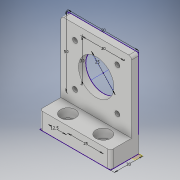
# Autodesk Inventor part: mirror-bracket
Saved by Autodesk Inventor 2017 (Build 210142000, 142)
## iProperties
Created: 2022-08-02
Part Number: mirror-bracket
Material: Generic
Document SubType Name: Modeling
Designer: Nikita
Density: 1 g/cm^3
Appearance: Default
Author: Nikita
Autodesk Inventor part; units mm, degrees
ref_plane "YZ Plane" through (0, 0, 0) normal (1, 0, 0) x (0, 1, 0)
ref_plane "XY Plane" through (0, 0, 0) normal (0, 0, 1) x (1, 0, 0)
sketch "Sketch1" plane through (0, 0, 0) normal (0, 0, 1) x (1, 0, 0)
  circle A0 centre (0, 0) radius 12.5
  line L0 (25, -25) -> (-25, -25)
  line L1 (-25, -25) -> (-25, 25)
  line L2 (-25, 25) -> (25, 25)
  line L3 (25, 25) -> (25, -25)
  line L4 (25, -25) -> (-25, 25) construction
  line L5 (-25, -25) -> (25, 25) construction
  point P0 (-15, 15)
  point P1 (15, 15)
  point P2 (-15, -15)
  point P3 (15, -15)
  dimension "d0" = 25
  dimension "d1" = 50
  dimension "d2" = 50
  dimension "d5" = 30
  dimension "d8" = 30
  constraints: 12 end point, 2 horizontal, 2 midpoint, 2 parallel, 1 centre point, 1 coincident, 1 perpendicular, 1 vertical, 3 other
  measures "d0" diameter of A0
  measures "d1" distance of L1.end L2.end
  measures "d2" distance of L0.end L1.end
  measures "d5" distance of point (-15, 15) point (15, 15)
  measures "d8" distance of point (-15, 15) point (-15, -15)
extrude "Extrusion1" add sketch "Sketch1" along normal blind 5
hole "Hole1" at (-15, 15, 0) at (15, 15, 0) at (-15, -15, 0) at (15, -15, 0) direction (0, 0, 1) diameter 3.5 end through all
ref_plane "Work Plane1" through (0, -37, 0) normal (0, 1, 0) x (-1, 0, 0)
sketch "Sketch2" plane through (0, -37, 0) normal (0, 1, 0) x (-1, 0, 0)
  line L0 (-25, 0) -> (25, 0) projected
  line L1 (-25, 0) -> (-25, 5) projected
  line L2 (25, 0) -> (-25, 0)
  line L3 (-25, 0) -> (-25, 20)
  line L4 (-25, 20) -> (25, 20)
  line L5 (25, 20) -> (25, 0)
  point P0 (0, 0)
  point P1 (12.5, 12.5)
  point P2 (-12.5, 12.5)
  dimension "d21" = 20
  dimension "d24" = 25
  dimension "d46" = 12.5
  constraints: 8 end point, 2 horizontal, 2 parallel, 1 perpendicular, 1 other
  measures "d21" distance of L0.start L3.end
  measures "d24" distance of point (12.5, 12.5) point (-12.5, 12.5)
  measures "d46" distance from line of L5 point (12.5, 12.5)
extrude "Extrusion2" add sketch "Sketch2" along normal up to surface (12 mm away)
hole "Hole2" at (12.5, -37, 12.5) at (-12.5, -37, 12.5) direction (0, 1, 0) diameter 6.5 end through all
fillet "Fillet1" radius 2 4 edges at (25, 25, 2.5) (-25, 25, 2.5) (25, -31, 20) (-25, -31, 20)
sketch "Sketch5" plane through (-25, -25, 5) normal (0, 1, 0) x (1, 0, 0)
  point P0 (25, 5)
  point P1 (12.5, -7.5)
  point P2 (37.5, -7.5)
hole "Hole4" at (-12.5, -25, 12.5) at (12.5, -25, 12.5) direction (0, -1, 0) diameter 10.5 depth 6.2
body "Solid1"
